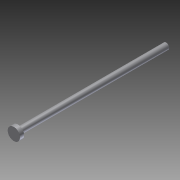
# Autodesk Inventor part: Plunger
Saved by Autodesk Inventor 2012 (Build 160160000, 160)
## iProperties
Created: 2011-09-11
Part Number: Plunger
Material: Default
Document SubType Name: Modeling
Designer: Ian Walters
Density: 1 g/cm^3
Author: Ian Walters
Autodesk Inventor part; units mm, degrees
ref_plane "YZ Plane" through (0, 0, 0) normal (1, 0, 0) x (0, 1, 0)
ref_plane "XZ Plane" through (0, 0, 0) normal (0, 1, 0) x (-1, 0, 0)
ref_plane "XY Plane" through (0, 0, 0) normal (0, 0, 1) x (1, 0, 0)
sketch "Sketch1" plane through (0, 0, 0) normal (0, 0, 1) x (1, 0, 0)
  circle A0 centre (0, 0) radius 9.525
  dimension "d0" = 19.05
  constraints: 1 centre point, 1 coincident
  measures "d0" diameter of A0
extrude "Extrusion1" add sketch "Sketch1" along normal mid plane 457.2
sketch "Sketch2" plane through (0, 0, 228.6) normal (0, 0, 1) x (1, 0, 0)
  circle A0 centre (0, 0) radius 9.525 projected
  circle A1 centre (0, 0) radius 19.05
  dimension "d3" = 38.1
  constraints: 1 centre point, 1 coincident
  measures "d3" diameter of A1
extrude "Extrusion2" add sketch "Sketch2" along normal blind 12.7 contours A0 | A1
body "Solid1"
